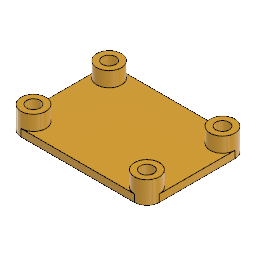
dcdc_carrier v1 (Autodesk Fusion 360 design; units mm, degrees)
Autodesk Fusion 360 part; units mm, degrees
sketch "Sketch1" plane through (0, 0, 0) normal (0, 0, 1) x (1, 0, 0)
  line L0 (22.86, -15.24) -> (-22.86, -15.24) construction
  line L1 (-22.86, -15.24) -> (-22.86, 15.24) construction
  line L2 (-22.86, 15.24) -> (22.86, 15.24) construction
  line L3 (22.86, 15.24) -> (22.86, -15.24) construction
  line L4 (22.86, -15.24) -> (-22.86, 15.24) construction
  line L5 (-22.86, -15.24) -> (22.86, 15.24) construction
  circle A0 centre (22.86, 15.24) radius 5
  circle A1 centre (22.86, -15.24) radius 5
  circle A2 centre (-22.86, -15.24) radius 5
  circle A3 centre (-22.86, 15.24) radius 5
  line L6 (-22.86, 20.24) -> (22.86, 20.24)
  line L7 (-27.86, 15.24) -> (-27.86, -15.24)
  line L8 (27.86, 15.24) -> (27.86, -15.24)
  line L9 (-22.86, -20.24) -> (22.86, -20.24)
  circle A4 centre (22.86, 15.24) radius 2.7
  circle A5 centre (-22.86, 15.24) radius 2.7
  circle A6 centre (-22.86, -15.24) radius 2.7
  circle A7 centre (22.86, -15.24) radius 2.7
  dimension "d1" = 45.72
  dimension "d2" = 30.48
  dimension "d3" = 10
  dimension "d4" = 10
  dimension "d5" = 10
  dimension "d6" = 10
  dimension "d12" = 5.4
  dimension "d13" = 5.4
  dimension "d14" = 5.4
  dimension "d15" = 5.4
  constraint perpendicular L0 L1
  constraint parallel L0 L2
  constraint parallel L1 L3
  constraint horizontal L0
  constraint coincident L4 origin
  constraint coincident L5 origin
  constraint coincident L2.end L3.start
  constraint coincident L0.start L3.end
  constraint coincident L0.end L1.start
  constraint coincident L1.end L2.start
  constraint coincident A3 L6.start
  constraint coincident A0 L6.end
  constraint tangent A0 L6
  constraint coincident A3 L7.start
  constraint coincident A2 L7.end
  constraint tangent A2 L7
  constraint coincident A0 L8.start
  constraint coincident A1 L8.end
  constraint tangent A1 L8
  constraint coincident A2 L9.start
  constraint tangent A2 L9
  constraint coincident A1 L9.end
  constraint tangent A1 L9
  constraint tangent A0 L8
  constraint tangent A3 L6
  constraint tangent A3 L7
  constraint concentric A3 A5
  constraint concentric A2 A6
  constraint concentric A1 A7
  measures "d1" distance of L1.end L2.end
  measures "d2" distance of L0.end L1.end
  measures "d3" diameter of A0
  measures "d4" diameter of A1
  measures "d5" diameter of A2
  measures "d6" diameter of A3
  measures "d12" diameter of A4
  measures "d13" diameter of A5
  measures "d14" diameter of A6
  measures "d15" diameter of A7
extrude "Extrude1" add sketch "Sketch1" along normal blind 3 contours A0 | A0 A1 A2 A3 L6 L7 L8 L9 | A1 | A3 | A2 | A4 | A5 | A6 | A7
extrude "Extrude2" add sketch "Sketch1" along normal blind 6 from surface at 3 contours A0 | A1 | A3 | A2 | A4 | A5 | A6 | A7
extrude "Extrude3" cut sketch "Sketch1" against normal blind 7 from surface at 9 contours A4 | A5 | A6 | A7
equation "d4 = d3"
equation "d5 = d3"
equation "d6 = d3"
equation "d13 = d12"
equation "d14 = d12"
equation "d15 = d12"
